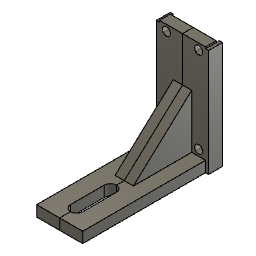
Bracket1 v5 (Autodesk Fusion 360 design; units mm, degrees)
Autodesk Fusion 360 part; units mm, degrees
sketch "Sketch1" plane through (0, 0, 0) normal (0, 1, 0) x (1, 0, 0)
  line L0 (15, -87.067) -> (0, -87.067) construction
  line L1 (15, -87.067) -> (25, -87.067) construction
  line L2 (25, -87.067) -> (25, 2.933) construction
  line L3 (25, 2.933) -> (15, 2.933) construction
  line L4 (15, 2.933) -> (15, -87.067) construction
  line L5 (0, -2) -> (-8.8435, -2) construction
  line L6 (-8.8435, -2) -> (-8.8435, -50) construction
  line L7 (-8.8435, -50) -> (0, -50) construction
  line L8 (0, -50) -> (0, -2) construction
  line L9 (-4, -54) -> (-4, -76)
  arc A0 (-4, -76) -> (4, -76) centre (0, -76) ccw
  line L10 (4, -76) -> (4, -54)
  arc A1 (4, -54) -> (-4, -54) centre (0, -54) ccw
  line L11 (0, -50) -> (0, -80) construction
  line L12 (0, -50) -> (30, -50) construction
  line L13 (0, -87.067) -> (15, -87.067)
  line L14 (15, -87.067) -> (15, -0.067)
  line L15 (15, -0.067) -> (0, -0.067)
  line L16 (0, -0.067) -> (0, -87.067)
  dimension "d9" = 90
  dimension "d10" = 48
  dimension "d11" = 30
  dimension "d12" = 90
  dimension "d13" = 8
  dimension "d21" = 15
  dimension "d22" = 87
  constraint horizontal L1
  constraint vertical L2
  constraint horizontal L3
  constraint vertical L4
  constraint horizontal L5
  constraint vertical L6
  constraint horizontal L7
  constraint vertical L8
  constraint tangent L9 A0
  constraint tangent A0 L10
  constraint parallel L9 L10
  constraint tangent L10 A1
  constraint tangent L9 A1
  constraint midpoint L7.end A1
  constraint midpoint A0 L11.end
  constraint horizontal L13
  constraint vertical L14
  constraint horizontal L15
  constraint vertical L16
  measures "d9" distance of L0.start L3.end
  measures "d10" distance of L5.start L7.end
  measures "d11" distance of L7.end L11.end
  measures "d12" angle of L11 L12
  measures "d13" diameter of A0
  measures "d21" distance of L0.end L0.start
  measures "d22" distance of L0.end L15.end
extrude "Extrude1" add sketch "Sketch1" along normal blind 7 contours A0 L10 A1 L13 L14 L15 L16 makes body 1
sketch "Sketch2" plane through (0, 0, 0) normal (0, 0, 1) x (1, 0, 0)
  circle A0 centre (10.5, 67) radius 2.65
  line L0 (0, 7) -> (15, 7)
  line L1 (15, 7) -> (15, 71)
  line L2 (15, 71) -> (0, 71)
  line L3 (0, 71) -> (0, 7)
  circle A1 centre (10.5, 11) radius 2.65
  dimension "d16" = 5.3
  dimension "d23" = 15
  dimension "d24" = 64
  dimension "d25" = 10.5
  dimension "d26" = 5.3
  constraint horizontal L0
  constraint vertical L1
  constraint horizontal L2
  constraint vertical L3
  measures "d16" diameter of A0
  measures "d23" distance of L0.start L0.end
  measures "d24" distance of L0.start L2.end
  measures "d25" distance of A0.centre L3
  measures "d26" diameter of A1
sketch "Sketch4" plane through (0, 0, 0) normal (0, 0, 1) x (1, 0, 0)
  line L0 (17, 70) -> (15, 70)
  line L1 (15, 70) -> (15, 0)
  line L2 (15, 0) -> (17, 0)
  line L3 (17, 0) -> (17, 70)
  dimension "d33" = 2
  constraint horizontal L0
  constraint vertical L1
  constraint horizontal L2
  constraint vertical L3
  measures "d33" distance of L0.start L0.end
extrude "Extrude2" add sketch "Sketch2" along normal blind 7 separate body makes body 2
extrude "Extrude3" add sketch "Sketch4" along normal blind 6 and the other way blind 3 from surface at 1 bodies 1 2
sketch "Sketch5" plane through (0, 0, 0) normal (1, 0, 0) x (0, 0, -1)
  line L0 (-7, 42) -> (-7, 7)
  line L1 (-7, 7) -> (-45, 7)
  line L2 (-45, 7) -> (-7, 42)
  constraint vertical L0
  constraint perpendicular L0 L1
extrude "Extrude4" add sketch "Sketch5" along normal blind 6 bodies 1
mirror "Mirror2" about plane through (0, 0, 0) normal (1, 0, 0) of bodies 1 makes body 3
combine "Combine1" operation add target body 1 tool bodies 3 keep tools result as body 4 in component "Component"
component "Component" placed x (1, 0, 0) y (0, 1, 0) z (0, 0, 1) at (0, 0, 0)
